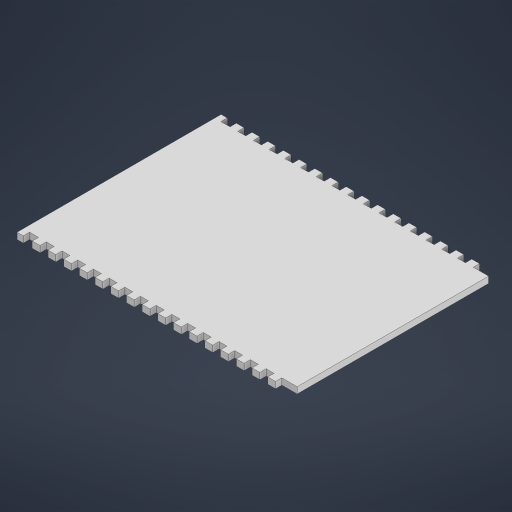
# Autodesk Inventor part: BodenWand
Saved by Autodesk Inventor 2023 (Build 270158030, 158C)
## iProperties
Created: 2022-06-21
Part Number: BodenWand
Material: Generic
Document SubType Name: Modeling
Designer: Simon
Density: 1 g/cm^3
Appearance: Default
Author: Simon
Autodesk Inventor part; units mm, degrees
ref_plane "YZ Plane" through (0, 0, 0) normal (1, 0, 0) x (0, 1, 0)
ref_plane "XZ Plane" through (0, 0, 0) normal (0, 1, 0) x (-1, 0, 0)
ref_plane "XY Plane" through (0, 0, 0) normal (0, 0, 1) x (1, 0, 0)
sketch "Sketch1" plane through (0, 0, 0) normal (0, 1, 0) x (-1, 0, 0)
  line L0 (9.7032, 0) -> (5.7032, 0)
  line L1 (5.7032, 0) -> (5.7032, -4)
  line L2 (5.7032, -4) -> (9.7032, -4)
  line L3 (9.7032, -4) -> (9.7032, 0)
  line L4 (0, 0) -> (-5, 0)
  line L5 (-5, 0) -> (-5, -4)
  line L6 (-5, -4) -> (0, -4)
  line L7 (0, -4) -> (0, 0)
  line L8 (-10, 0) -> (-15, 0)
  line L9 (-15, 0) -> (-15, -4)
  line L10 (-15, -4) -> (-10, -4)
  line L11 (-10, -4) -> (-10, 0)
  line L12 (-20, 0) -> (-25, 0)
  line L13 (-25, 0) -> (-25, -4)
  line L14 (-25, -4) -> (-20, -4)
  line L15 (-20, -4) -> (-20, 0)
  line L16 (-30, 0) -> (-35, 0)
  line L17 (-35, 0) -> (-35, -4)
  line L18 (-35, -4) -> (-30, -4)
  line L19 (-30, -4) -> (-30, 0)
  line L20 (-40, 0) -> (-45, 0)
  line L21 (-45, 0) -> (-45, -4)
  line L22 (-45, -4) -> (-40, -4)
  line L23 (-40, -4) -> (-40, 0)
  line L24 (-50, 0) -> (-55, 0)
  line L25 (-55, 0) -> (-55, -4)
  line L26 (-55, -4) -> (-50, -4)
  line L27 (-50, -4) -> (-50, 0)
  line L28 (-60, 0) -> (-65, 0)
  line L29 (-65, 0) -> (-65, -4)
  line L30 (-65, -4) -> (-60, -4)
  line L31 (-60, -4) -> (-60, 0)
  line L32 (-70, 0) -> (-75, 0)
  line L33 (-75, 0) -> (-75, -4)
  line L34 (-75, -4) -> (-70, -4)
  line L35 (-70, -4) -> (-70, 0)
  line L36 (-80, 0) -> (-85, 0)
  line L37 (-85, 0) -> (-85, -4)
  line L38 (-85, -4) -> (-80, -4)
  line L39 (-80, -4) -> (-80, 0)
  line L40 (-90, 0) -> (-95, 0)
  line L41 (-95, 0) -> (-95, -4)
  line L42 (-95, -4) -> (-90, -4)
  line L43 (-90, -4) -> (-90, 0)
  line L44 (-100, 0) -> (-105, 0)
  line L45 (-105, 0) -> (-105, -4)
  line L46 (-105, -4) -> (-100, -4)
  line L47 (-100, -4) -> (-100, 0)
  line L48 (-110, 0) -> (-115, 0)
  line L49 (-115, 0) -> (-115, -4)
  line L50 (-115, -4) -> (-110, -4)
  line L51 (-110, -4) -> (-110, 0)
  line L52 (-120, 0) -> (-125, 0)
  line L53 (-125, 0) -> (-125, -4)
  line L54 (-125, -4) -> (-120, -4)
  line L55 (-120, -4) -> (-120, 0)
  line L56 (-130, 0) -> (-135, 0)
  line L57 (-135, 0) -> (-135, -4)
  line L58 (-135, -4) -> (-130, -4)
  line L59 (-130, -4) -> (-130, 0)
  line L60 (-140, 0) -> (-145, 0)
  line L61 (-145, 0) -> (-145, -4)
  line L62 (-145, -4) -> (-140, -4)
  line L63 (-140, -4) -> (-140, 0)
  line L64 (-150, 0) -> (-155, 0)
  line L65 (-155, 0) -> (-155, -4)
  line L66 (-155, -4) -> (-150, -4)
  line L67 (-150, -4) -> (-150, 0)
  line L68 (0, -65) -> (-164, -65)
  line L69 (-164, -65) -> (-164, -4)
  line L70 (-164, -4) -> (0, -4)
  line L71 (0, -65) -> (9.7032, -65)
  line L72 (9.7032, -65) -> (9.7032, -4)
  line L73 (9.7032, -4) -> (0, -4)
  dimension "d4" = 5
  dimension "d5" = 4
  dimension "d6" = 10
  constraints: 146 end point, 6 horizontal, 5 parallel, 4 perpendicular, 1 collinear, 122 other
  measures "d4" distance of L6.end L5.end
  measures "d5" distance of L5.end L4.end
  measures "d6" distance of L5.end L9.end
extrude "Extrusion1" add sketch "Sketch1" along normal blind 4
move faces "Move1" translate (0.75, 0, 0) faces at (164, 1.3333, -24.3333)
mirror "Mirror1" about plane through (164, 0, -65) normal (0, 0, -1) of "Extrusion1"
move faces "Move2" translate (0.75, 0, 0) faces at (164, 1.3333, -105.6667)
body "Solid1"
